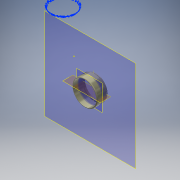
# Autodesk Inventor part: adaptador_cono
Saved by Autodesk Inventor 2019 (Build 230136000, 136)
## iProperties
Created: 2019-01-08
Part Number: adaptador_cono
Material: PET Plastic
Document SubType Name: Modeling
Designer: jmc
Density: 1.541 g/cm^3
Appearance: Smooth - Ash
Author: jmc
Autodesk Inventor part; units mm, degrees
ref_plane "YZ Plane" through (0, 0, 0) normal (1, 0, 0) x (0, 1, 0)
ref_plane "XZ Plane" through (0, 0, 0) normal (0, 1, 0) x (-1, 0, 0)
ref_plane "XY Plane" through (0, 0, 0) normal (0, 0, 1) x (1, 0, 0)
ref_plane "Work Plane1" through (67.8466, -36.9116, -13.6178) normal (0, 0, -1) x (1, 0, 0)
sketch "Sketch1" plane through (67.8466, -36.9116, -13.6178) normal (0, 0, -1) x (1, 0, 0)
  circle A0 centre (-25.3126, -0.0255) radius 25 projected
  circle A1 centre (-25.3126, -0.0255) radius 25.15
  circle A2 centre (-25.3126, -0.0255) radius 27.15
  point P0 (-67.8466, -36.9116)
  dimension "d8" = 0.15
  dimension "d9" = 2
  dimension "d26" = 54.3
  constraints: 2 centre point, 2 coincident
  measures "d8" radial gap between concentric circles of A0 A1
  measures "d9" radial gap between concentric circles of A1 A2
  measures "d26" diameter of A2
extrude "Extrusion2" add sketch "Sketch1" along normal mid plane 20 contours A2
fillet "Fillet3" radius 2 1 edges at (15.384, -36.8861, -3.6178)
sketch "Sketch3" plane through (42.534, -36.8861, -23.6178) normal (0, 0, -1) x (-1, 0, 0)
  line L0 (-31.2994, 0) -> (31.4368, 0) construction
  line L1 (0.0687, 33.0391) -> (0.0687, -31.9659) construction
  point P0 (42.534, 36.8861)
  constraints: 4 end point, 1 horizontal, 1 vertical
ref_plane "Work Plane3" through (73.8334, -36.8861, -23.6178) normal (0, 1, 0) x (-1, 0, 0)
ref_plane "Work Plane2" through (42.539, -36.9116, -12.6178) normal (0, 0, 1) x (-1, 0, 0)
sketch "Sketch4" plane through (73.8334, -36.8861, -23.6178) normal (0, 1, 0) x (-1, 0, 0)
  line L0 (6.1494, 20) -> (6.1494, 0) construction
  line L1 (56.4494, 20) -> (56.4494, 0) construction
  line L2 (4.1494, 0) -> (6.1494, -2)
  line L3 (6.1494, -2) -> (6.1494, -4)
  line L4 (6.1494, -4) -> (8.1494, -4)
  line L5 (31.2994, 0.6713) -> (31.2994, 28.2514) construction
  line L6 (31.2994, 28.2514) -> (31.2994, -7.4559) construction
  line L7 (8.1494, -0.2025) -> (6.2913, -0.2025)
  line L8 (4.1494, 0) -> (6.1496, 0)
  line L9 (4.1494, 0) -> (6.1494, 0) construction
  line L10 (6.2911, 0) -> (6.9778, 0) construction
  line L11 (6.2913, -0.2025) -> (6.1496, -0.2025)
  line L12 (6.1496, -0.2025) -> (6.1496, 0)
  line L13 (8.2994, -0.2025) -> (8.2994, 19.7975) construction
  line L14 (8.1494, -0.2025) -> (8.2994, -0.2025)
  line L15 (8.2994, -0.2025) -> (8.2994, -4)
  line L16 (8.2994, -4) -> (8.1494, -4)
  point P0 (73.8334, 23.6178)
  dimension "d18" = 2
  constraints: 31 end point, 6 horizontal, 4 vertical, 2 point on line, 1 collinear, 2 other
  measures "d18" distance of L2.end L3.end
revolve "Revolution1" add sketch "Sketch4" angle 360 about axis through (42.534, -36.8861, 4.6336) along (0, 0, -1)
fillet "Fillet5" radius 2 2 edges at (17.384, -36.8861, -25.6178) (15.384, -36.8861, -23.6178)
ref_plane "Work Plane4" through (42.534, -36.8861, -15.6178) normal (0, 0, -1) x (0, 1, 0)
ref_plane "Work Plane5" through (42.534, -36.8861, -15.6178) normal (0, 0, -1) x (0, 1, 0)
sketch "Sketch6" plane through (42.534, -36.8861, -15.6178) normal (0, 0, -1) x (0, 1, 0)
  line L0 (-5, -31.75) -> (5, -31.75) projected
  line L1 (5, 31.75) -> (-5, 31.75) projected
  line L2 (-31.75, 5) -> (-31.75, -5) projected
  line L3 (31.75, -5) -> (31.75, 5) projected
  line L4 (1.7812, -31.75) -> (7.9821, -31.75)
  line L5 (31.75, -7.9821) -> (31.75, 7.9821)
  line L6 (7.9821, 31.75) -> (-7.9821, 31.75)
  line L7 (-31.75, 7.9821) -> (-31.75, -7.9821)
  line L8 (-7.9821, -31.75) -> (-1.7661, -31.75)
  circle A0 centre (0, 0) radius 27.15 projected
  arc A1 (-31.75, -7.9821) -> (-7.9821, -31.75) centre (0, 0) ccw
  arc A2 (-7.9821, 31.75) -> (-31.75, 7.9821) centre (0, 0) ccw
  arc A3 (7.9821, -31.75) -> (31.75, -7.9821) centre (0, 0) ccw
  arc A4 (31.75, 7.9821) -> (7.9821, 31.75) centre (0, 0) ccw
  point P0 (36.8861, -42.534)
  point P1 (-31.75, -31.75)
  constraints: 10 end point, 8 point on circle, 4 centre point, 3 perpendicular, 3 point on line, 1 coincident, 1 horizontal
extrude "Extrusion4" add sketch "Sketch6" along normal blind 2
equation "\"d8\" = HOLE_TOLERANCE"
equation "\"HOLE_TOLERANCE\" = 0.15"
body "Solid2"
